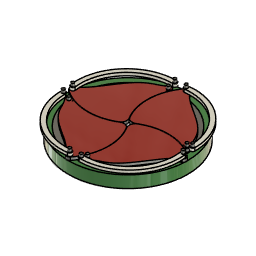
Iris Slider v1 (Autodesk Fusion 360 design; units mm, degrees)
Autodesk Fusion 360 part; units mm, degrees
sketch "Sketch1" plane through (0, 0, 0) normal (0, 0, 1) x (1, 0, 0)
  circle A0 centre (0, 0) radius 100
  circle A1 centre (0, 0) radius 90
  circle A2 centre (0, 0) radius 80
  dimension "d1" = 200
  dimension "d2" = 180
  dimension "d3" = 160
  constraint coincident A0.centre A1.centre
  measures "d1" diameter of A0
  measures "d2" diameter of A1
  measures "d3" diameter of A2
extrude "Extrude1" add sketch "Sketch1" against normal blind 20 contours A0 makes body 1 in component "base1"
extrude "Extrude1'" add sketch "Sketch1" against normal blind 20 separate body contours A1 makes body 2 in component "base2"
sketch "Sketch2" plane through (0, 0, 0) normal (0, 0, 1) x (1, 0, 0)
  circle A0 centre (0, 0) radius 80
  circle A1 centre (0, 0) radius 90
  circle A2 centre (0, 0) radius 90
  circle A3 centre (0, 0) radius 100
  arc A4 (0, 100) -> (0, 0) centre (62.45, 50) ccw
  arc A5 (100, 0) -> (0, 0) centre (50, -62.45) ccw
  circle A6 centre (2.4267, 94.969) radius 5
  circle A7 centre (83.5469, 15.65) radius 5
  spline S0 degree 5 poles (6.7933, 97.4048) (7.2781, 96.5358) (8.3865, 94.784) (10.4657, 92.115) (14.0581, 88.4719) (19.8153, 83.7666) (26.6651, 78.8976) (34.3503, 73.856) (42.5105, 68.6417) (50.6765, 63.2675) (58.358, 57.7564) (65.1167, 52.1397) (70.652, 46.4562) (74.8749, 40.7504) (78.0282, 35.0733) (80.6973, 29.4793) (82.9878, 25.1101) (85.0539, 21.9095) (86.6213, 19.8117) (87.4525, 18.7719) knots 0 0 0 0 0 0 0.066667 0.133333 0.2 0.266667 0.333333 0.4 0.466667 0.533333 0.6 0.666667 0.733333 0.8 0.866667 0.933333 1 1 1 1 1 1
  line L0 (79.4483, 28.7856) -> (95.4567, 8.7581)
  line L1 (2.7453, 104.6615) -> (10.8413, 90.1481)
  circle A8 centre (2.4267, 94.969) radius 2.5
  circle A9 centre (83.5469, 15.65) radius 2.5
  point P0 (33.1146, 74.6949)
  point P1 (73.3851, 42.5507)
  dimension "d8" = 80
  dimension "d10" = -90
  dimension "d11" = 5
  dimension "d12" = 5
  constraint coincident A3 A4.start
  constraint coincident A0.centre A1.centre
  constraint vertical A0.centre A4.start
  constraint tangent A4 A6
  constraint tangent A3 A6
  constraint tangent A1 A6
  constraint tangent A1 A7
  constraint tangent A5 A7
  constraint tangent A0 A7
  constraint coincident A6 S0.start
  constraint coincident A7 S0.end
  constraint midpoint S0.end L0
  constraint midpoint S0.start L1
  constraint tangent A7 L0
  constraint tangent A6 L1
  constraint concentric A6 A8
  constraint concentric A7 A9
  measures "d8" radius of A4
  measures "d11" diameter of A8
  measures "d12" diameter of A9
extrude "Extrude1''" add sketch "Sketch2" along normal blind 5 separate body contours A0 A4 A5 | A0 A1 A2 A4 A7 S0 | A7 | A1 A2 A4 A6 | A1 A2 A6 S0 | A6 picked at (11.6715, 43.094) makes body 3 in component "shutter1"
sketch "Sketch3" plane through (0, 0, 5) normal (0, 0, 1) x (-1, 0, 0)
  circle A0 centre (-2.4267, -94.969) radius 2.5
  circle A1 centre (-83.5469, -15.65) radius 2.5
  arc A2 (1.5748, -97.9669) -> (0, 0) centre (-62.45, -50) ccw
  arc A3 (-79.0833, -12.0763) -> (0, 0) centre (-50, 62.45) ccw
  arc A4 (-79.0833, -12.0763) -> (-78.6323, -14.7294) centre (0, 0) ccw
  arc A5 (-78.6323, -14.7294) -> (-87.4525, -18.7719) centre (-83.5469, -15.65) ccw
  spline S0 degree 5 poles (-87.4525, -18.7719) (-86.6213, -19.8117) (-85.0539, -21.9095) (-82.9878, -25.1101) (-80.6973, -29.4793) (-78.0282, -35.0733) (-74.8749, -40.7504) (-70.652, -46.4562) (-65.1167, -52.1397) (-58.358, -57.7564) (-50.6765, -63.2675) (-42.5105, -68.6417) (-34.3503, -73.856) (-26.6651, -78.8976) (-19.8153, -83.7666) (-14.0581, -88.4719) (-10.4657, -92.115) (-8.3865, -94.784) (-7.2781, -96.5358) (-6.7933, -97.4048) knots -1 -1 -1 -1 -1 -1 -0.933333 -0.866667 -0.8 -0.733333 -0.666667 -0.6 -0.533333 -0.466667 -0.4 -0.333333 -0.266667 -0.2 -0.133333 -0.066667 0 0 0 0 0 0
  arc A6 (-6.7933, -97.4048) -> (1.5748, -97.9669) centre (-2.4267, -94.969) ccw
  circle A7 centre (-83.5469, -15.65) radius 2.5
  circle A8 centre (-2.4267, -94.969) radius 2.5
  arc A9 (-6.7933, -97.4048) -> (1.5748, -97.9669) centre (-2.4267, -94.969) ccw
  spline S1 degree 5 poles (-6.7933, -97.4048) (-7.2781, -96.5358) (-8.3865, -94.784) (-10.4657, -92.115) (-14.0581, -88.4719) (-19.8153, -83.7666) (-26.6651, -78.8976) (-34.3503, -73.856) (-42.5105, -68.6417) (-50.6765, -63.2675) (-58.358, -57.7564) (-65.1167, -52.1397) (-70.652, -46.4562) (-74.8749, -40.7504) (-78.0282, -35.0733) (-80.6973, -29.4793) (-82.9878, -25.1101) (-85.0539, -21.9095) (-86.6213, -19.8117) (-87.4525, -18.7719) knots 0 0 0 0 0 0 0.066667 0.133333 0.2 0.266667 0.333333 0.4 0.466667 0.533333 0.6 0.666667 0.733333 0.8 0.866667 0.933333 1 1 1 1 1 1
  arc A10 (-78.6323, -14.7294) -> (-87.4525, -18.7719) centre (-83.5469, -15.65) ccw
  arc A11 (-79.0833, -12.0763) -> (-78.6323, -14.7294) centre (0, 0) ccw
  arc A12 (-79.0833, -12.0763) -> (0, 0) centre (-50, 62.45) ccw
  arc A13 (1.5748, -97.9669) -> (0, 0) centre (-62.45, -50) ccw
  circle A14 centre (-93.5, -15) radius 3.75
  circle A15 centre (-93.5, -15) radius 2.5
  circle A16 centre (-2.4267, -94.969) radius 3.75
  arc A17 (-97.25, -15) -> (-2.4267, -98.719) centre (-12.8808, -15) ccw
  arc A18 (-89.75, -15) -> (-2.4267, -91.219) centre (-12.825, -15) ccw
  dimension "d15" = 7.5
  dimension "d16" = 5
  dimension "d17" = 15
  dimension "d18" = 93.5
  dimension "d19" = 7.5
  constraint concentric A14 A15
  constraint concentric A8 A16
  constraint coincident A14 A17.start
  constraint coincident A16 A17.end
  constraint vertical A0.centre A17.end
  constraint horizontal A14.centre A17.start
  constraint tangent A14 A17
  constraint tangent A14 A18
  constraint coincident A14 A18.start
  constraint coincident A16 A18.end
  constraint vertical A0.centre A18.end
  constraint horizontal A14.centre A18.start
  measures "d15" diameter of A14
  measures "d16" diameter of A15
  measures "d17" vertical distance of A2.end A14.centre
  measures "d18" horizontal distance of A2.end A14.centre
  measures "d19" diameter of A16
extrude "Extrude1'''" add sketch "Sketch3" along normal blind 5 separate body contours S0 A6 A9 S1 A14 A17 A18 | S0 A6 A9 S1 A16 A17 A18 | A14 | A16 A18 picked at (-2.6686, -98.287) makes body 4 in component "link1"
extrude "Extrude1''''" add sketch "Sketch3" along normal blind 10 separate body contours A15 makes body 5
fillet "Fillet1" radius 10 1 edges at (0, 0, 2.5) on bodies 3 in component "shutter1"
copy_body "CutPasteBodies1" bodies 5 removing the originals makes body 6 in component "base1"
extrude "Extrude2" add sketch "Sketch3" along normal blind 10 separate body contours A0 A8 makes body 7
copy_body "CutPasteBodies1'" bodies 7 removing the originals makes body 8 in component "link1"
extrude "Extrude3" add sketch "Sketch3" along normal blind 5 separate body contours A1 A7 makes body 9
copy_body "CutPasteBodies1''" bodies 9 removing the originals makes body 10 in component "base2"
component_pattern "component pattern"
component_pattern "component pattern'"
pattern_circular "C-Pattern1" count 4 over 360 about axis through (0, 0, 0) along (0, 0, -1) of bodies 10 makes body 11 at (15.7746, -81.05, 8.3333) makes body 12 at (-84.6874, -17.8747, 6.6667) makes body 13 at (-17.8747, 84.6874, 6.6667) in component "base2"
pattern_circular "C-Pattern1'" count 4 over 360 about axis through (0, 0, 0) along (0, 0, -1) of bodies 6 makes body 14 at (15.1246, -91.0031, 11.6667) makes body 15 at (-91.0031, -15.1246, 11.6667) makes body 16 at (-15.1246, 91.0031, 11.6667) in component "base1"
component "shutter1" placed x (1, 0, 0) y (0, 1, 0) z (0, 0, 1) at (0, 0, 0)
component "link1" placed x (1, 0, 0) y (0, 1, 0) z (0, 0, 1) at (0, 0, 0)
component "base2" placed x (1, 0, 0) y (0, 1, 0) z (0, 0, 1) at (0, 0, 0)
component "base1" placed x (1, 0, 0) y (0, 1, 0) z (0, 0, 1) at (0, 0, 0)
component "link1" placed x (0, 1, 0) y (-1, 0, 0) z (0, 0, 1) at (0, 0, 0)
component "link1" placed x (-1, 0, 0) y (0, -1, 0) z (0, 0, 1) at (0, 0, 0)
component "link1" placed x (0, -1, 0) y (1, 0, 0) z (0, 0, 1) at (0, 0, 0)
component "shutter1" placed x (0, 1, 0) y (-1, 0, 0) z (0, 0, 1) at (0, 0, 0)
component "shutter1" placed x (-1, 0, 0) y (0, -1, 0) z (0, 0, 1) at (0, 0, 0)
component "shutter1" placed x (0, -1, 0) y (1, 0, 0) z (0, 0, 1) at (0, 0, 0)
